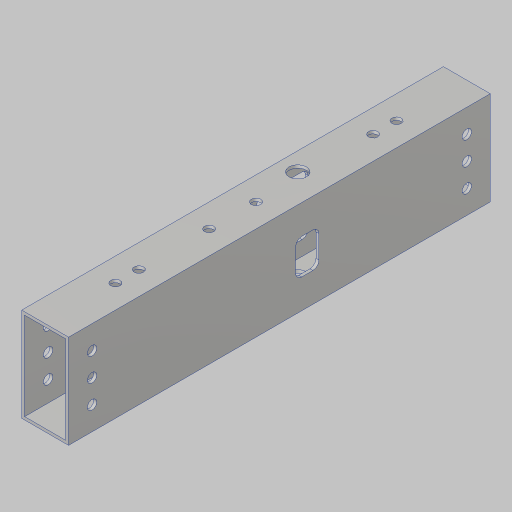
# Autodesk Inventor part: EL2-C-005
Saved by Autodesk Inventor 2023.5 (Build 275446000, 446)
## iProperties
RuleStatus: InUse
Created: 2025-01-11
Part Number: EL2-C-005
Material: Aluminum 6061
Document SubType Name: Modeling
Designer: brand
Mass: 304.185 g
Surface Area: 718.547 cm^2
Volume: 112.661 cm^3
Density: 2.7 g/cm^3
Appearance: Aluminum - Flat
AfterDocNew0: SHOW
AfterDocOpen0: SHOW
Author: brand
Autodesk Inventor part; units mm, degrees
ref_plane "YZ Plane" through (0, 0, 0) normal (1, 0, 0) x (0, 1, 0)
ref_plane "XZ Plane" through (0, 0, 0) normal (0, 1, 0) x (-1, 0, 0)
ref_plane "XY Plane" through (0, 0, 0) normal (0, 0, 1) x (1, 0, 0)
sketch "Sketch1" plane through (0, 0, 0) normal (0, 0, 1) x (1, 0, 0)
  line L0 (-12.7, -25.4) -> (12.7, -25.4)
  line L1 (12.7, -25.4) -> (12.7, 25.4)
  line L2 (12.7, 25.4) -> (-12.7, 25.4)
  line L3 (-12.7, 25.4) -> (-12.7, -25.4)
  line L4 (-12.7, -25.4) -> (12.7, 25.4) construction
  line L5 (12.7, -25.4) -> (-12.7, 25.4) construction
  line L6 (-11.1125, 23.8125) -> (11.1125, 23.8125)
  line L7 (11.1125, 23.8125) -> (11.1125, -23.8125)
  line L8 (11.1125, -23.8125) -> (-11.1125, -23.8125)
  line L9 (-11.1125, -23.8125) -> (-11.1125, 23.8125)
  point P0 (0, 0)
  dimension "width" = 25.4
  dimension "height" = 50.8
  dimension "thickness" = 1.5875
  constraints: 20 end point, 4 parallel, 2 midpoint, 2 perpendicular, 1 horizontal, 3 other
  measures "width" distance of L2.end L1.end
  measures "height" distance of L1.end L0.end
  measures "thickness" distance between parallel lines of L2 L6
extrude "Extrusion1" add sketch "Sketch1" along normal mid plane 228.6
sketch "Sketch2" plane through (-12.7, -25.4, 114.3) normal (-1, 0, 0) x (0, 0, 1)
  line L0 (-228.6, 0) -> (-228.6, 50.8) construction
  line L1 (-228.6, 50.8) -> (0, 50.8) construction
  line L2 (0, 50.8) -> (0, 0) construction
  line L3 (0, 0) -> (-228.6, 0) construction
  point P0 (-114.3, 25.4)
  point P1 (-215.9, 38.1)
  point P2 (-215.9, 25.4)
  point P3 (-215.9, 12.7)
  point P4 (-12.7, 38.1)
  point P5 (-12.7, 25.4)
  point P6 (-12.7, 12.7)
  point P7 (-228.6, 25.4)
  dimension "d5" = 12.7
  dimension "d6" = 12.7
  dimension "d7" = 12.7
  dimension "d8" = 12.7
  constraints: 4 horizontal alignment, 4 vertical alignment, 1 midpoint
  measures "d5" distance of point (-215.9, 38.1) point (-215.9, 25.4)
  measures "d6" distance of point (-215.9, 12.7) point (-215.9, 25.4)
  measures "d7" distance from line of L0 point (-215.9, 25.4)
  measures "d8" distance from line of L2 point (-12.7, 25.4)
hole "Block Mount Holes" at (-12.7, 12.7, -101.6) at (-12.7, 0, -101.6) at (-12.7, -12.7, -101.6) at (-12.7, 12.7, 101.6) at (-12.7, 0, 101.6) at (-12.7, -12.7, 101.6) direction (1, 0, 0) diameter 5.1054 end through all clearance for "Flat Head Machine Screw (82)" size "#10" standard "Ansi Unified Screw Threads"
sketch "Sketch4" plane through (-12.7, 25.4, 114.3) normal (0, 1, 0) x (1, 0, 0)
  line L0 (0, 228.6) -> (25.4, 228.6) projected
  line L1 (12.7, 177.8) -> (12.7, 50.8) construction
  point P0 (12.7, 114.3)
  point P1 (12.7, 228.6)
  point P2 (12.7, 190.5)
  point P3 (12.7, 38.1)
  point P4 (12.7, 114.3)
  dimension "d61" = 12.7
  dimension "d65" = 127
  dimension "d66" = 12.7
  constraints: 3 vertical alignment, 2 end point, 2 midpoint, 1 coincident, 1 vertical
  measures "d61" distance of point (12.7, 190.5) L1.start
  measures "d65" distance of L1.end L1.start
  measures "d66" distance of L1.end point (12.7, 38.1)
hole "Hole3" at (0, 25.4, 63.5) at (0, 25.4, -63.5) at (0, 25.4, -76.2) at (0, 25.4, 76.2) direction (0, -1, 0) diameter 5.1054 end through all clearance for "Flat Head Machine Screw (82)" size "#10" standard "Ansi Unified Screw Threads"
sketch "Sketch5" plane through (-12.7, -25.4, 114.3) normal (-1, 0, 0) x (0, 0, 1)
  line L0 (-153.67, 9.525) -> (-125.73, 9.525)
  line L1 (-125.73, 9.525) -> (-125.73, 41.275)
  line L2 (-125.73, 41.275) -> (-153.67, 41.275)
  line L3 (-153.67, 41.275) -> (-153.67, 9.525)
  line L4 (-228.6, 0) -> (-228.6, 50.8) projected
  point P0 (-114.3, 25.4)
  point P1 (-153.67, 25.4)
  point P2 (-228.6, 25.4)
  point P3 (-139.7, 9.525)
  point P4 (-139.7, 41.275)
  dimension "d37" = 31.75
  dimension "d38" = 27.94
  dimension "d78" = 25.4
  constraints: 8 end point, 4 midpoint, 2 parallel, 1 horizontal, 1 horizontal alignment, 1 perpendicular
  measures "d37" distance from line of L2 point (-139.7, 9.525)
  measures "d38" distance between parallel lines of L3 L1
  measures "d78" horizontal distance of point (-114.3, 25.4) point (-139.7, 41.275)
extrude "Extrusion2" cut sketch "Sketch5" against normal blind 1.5875
fillet "Fillet1" radius 3.302 4 edges at (-11.9062, -15.875, -39.37) (-11.9062, 15.875, -39.37) (-11.9062, 15.875, -11.43) (-11.9062, -15.875, -11.43)
sketch "Sketch6" plane through (-12.7, -25.4, 114.3) normal (0, -1, 0) x (1, 0, 0)
  line L0 (25.4, -228.6) -> (0, -228.6) projected
  line L1 (0, 0) -> (0, -228.6) projected
  line L2 (25.4, -228.6) -> (25.4, 0) construction
  point P0 (12.7, -114.3)
  point P1 (9.9314, -139.7)
  point P2 (12.7, -228.6)
  dimension "d63" = 9.9314
  dimension "d76" = 25.4
  constraints: 1 midpoint
  measures "d63" distance from line of L1 point (9.931, -139.7)
  measures "d76" vertical distance of point (12.7, -114.3) point (9.931, -139.7)
hole "Hole4" at (-2.7686, -25.4, -25.4) direction (0, 1, 0) diameter 9.525 end through all
sketch "Sketch7" plane through (12.7, -25.4, 114.3) normal (1, 0, 0) x (0, 0, -1)
  line L0 (228.6, 50.8) -> (228.6, 0) projected
  line L1 (135.7376, 34.925) -> (123.0376, 34.925)
  line L2 (123.0376, 34.925) -> (123.0376, 15.875)
  line L3 (123.0376, 15.875) -> (135.7376, 15.875)
  line L4 (135.7376, 15.875) -> (135.7376, 34.925)
  line L5 (135.7376, 34.925) -> (123.0376, 15.875) construction
  line L6 (123.0376, 34.925) -> (135.7376, 15.875) construction
  point P0 (114.3, 25.4)
  point P1 (129.3876, 25.4)
  point P2 (228.6, 25.4)
  dimension "d56" = 12.7
  dimension "d57" = 19.05
  dimension "d77" = 15.0876
  constraints: 12 end point, 3 midpoint, 2 parallel, 1 horizontal, 1 horizontal alignment, 1 perpendicular
  measures "d56" distance of L1.start L1.end
  measures "d57" distance of L1.end L2.end
  measures "d77" distance of point (114.3, 25.4) point (129.388, 25.4)
extrude "Extrusion3" cut sketch "Sketch7" against normal blind 1.5875
fillet "Fillet2" radius 3.302 4 edges at (11.9062, 9.525, -21.4376) (11.9062, -9.525, -21.4376) (11.9062, -9.525, -8.7376) (11.9062, 9.525, -8.7376)
sketch "Sketch8" plane through (-12.7, 25.4, 114.3) normal (0, 1, 0) x (1, 0, 0)
  circle A0 centre (9.9314, 139.7) radius 4.7625 construction
  circle A1 centre (12.7, 190.5) radius 2.5527 construction
  circle A2 centre (12.7, 50.8) radius 2.5527 construction
  circle A3 centre (12.7, 177.8) radius 2.5527 construction
  circle A4 centre (12.7, 38.1) radius 2.5527 construction
  line L0 (0, 228.6) -> (25.4, 228.6) construction
  line L1 (25.4, 228.6) -> (25.4, 0) construction
  line L2 (25.4, 0) -> (0, 0) construction
  line L3 (0, 0) -> (0, 228.6) construction
  point P0 (12.7, 114.3)
  point P1 (12.7, 114.3)
  point P2 (12.7, 88.9)
  dimension "d67" = 25.4
  dimension "d68" = 25.4
  constraints: 1 coincident, 1 vertical alignment
  measures "d67" distance of point (12.7, 88.9) point (12.7, 114.3)
  measures "d68" vertical distance of A0.centre point (12.7, 114.3)
hole "Hole5" at (0, 25.4, 0) at (0, 25.4, 25.4) direction (0, -1, 0) diameter 5.1054 end through all clearance for "Flat Head Machine Screw (82)" size "#10" standard "Ansi Unified Screw Threads"
equation "\"d6\" = d5"
equation "\"d8\" = d7"
body "Solid1"
